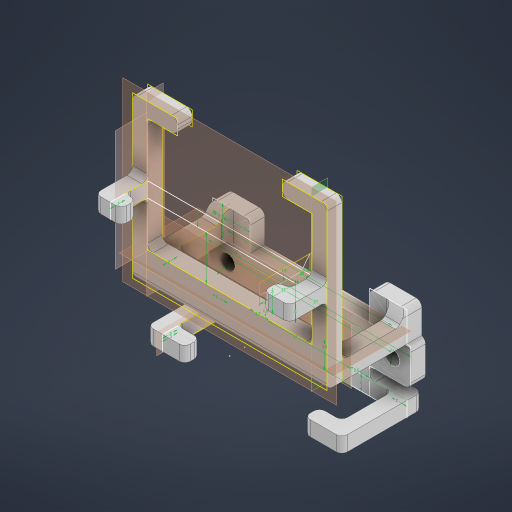
# Autodesk Inventor part: battery-stopper-3
Saved by Autodesk Inventor 2023.5 (Build 275446000, 446)
## iProperties
Created: 2025-02-09
Part Number: battery-stopper-3
Material: 一般
Document SubType Name: Modeling
Designer: IshiiLabHonda
Density: 1 g/cm^3
Appearance: 既定
Author: IshiiLabHonda
Autodesk Inventor part; units mm, degrees
ref_plane "YZ Plane" through (0, 0, 0) normal (1, 0, 0) x (0, 1, 0)
ref_plane "XZ Plane" through (0, 0, 0) normal (0, 1, 0) x (-1, 0, 0)
ref_plane "XY Plane" through (0, 0, 0) normal (0, 0, 1) x (1, 0, 0)
sketch "スケッチ1" plane through (0, 0, 0) normal (0, 0, 1) x (1, 0, 0)
  line L0 (0, 0) -> (0, 1.8035) construction
  line L1 (1.7104, 0) -> (0, 0) construction
  circle A0 centre (-11, 0) radius 1
  circle A1 centre (11, 0) radius 1
  line L2 (-13.5, 2.5) -> (13.5, 2.5)
  line L3 (13.5, 2.5) -> (13.5, -2.5)
  line L4 (13.5, -2.5) -> (-13.5, -2.5)
  line L5 (-13.5, -2.5) -> (-13.5, 2.5)
  line L6 (-13.5, 2.5) -> (13.5, -2.5) construction
  line L7 (13.5, 2.5) -> (-13.5, -2.5) construction
  circle A2 centre (-11, 0) radius 2.5 construction
  line L8 (-13, 6.5) -> (-8, 6.5)
  line L9 (-8, 6.5) -> (-8, 2.5)
  line L10 (-8, 2.5) -> (-13, 2.5)
  line L11 (-13, 2.5) -> (-13, 6.5)
  line L12 (-13, 6.5) -> (-8, 2.5) construction
  line L13 (-8, 6.5) -> (-13, 2.5) construction
  line L14 (-11, 6.5) -> (-11, 2.5)
  line L15 (13, 6.5) -> (8, 6.5)
  line L16 (8, 6.5) -> (8, 2.5)
  line L17 (13, 2.5) -> (13, 6.5)
  line L18 (13, 6.5) -> (8, 2.5) construction
  line L19 (8, 6.5) -> (13, 2.5) construction
  line L20 (11, 6.5) -> (11, 2.5)
  line L21 (-5.5, -2.5) -> (-5.5, -6)
  line L22 (-8, -2.5) -> (-8, -6)
  line L23 (8, -2.5) -> (8, -6)
  line L24 (5.5, -2.5) -> (5.5, -6)
  line L25 (8, -6) -> (5.5, -6)
  line L26 (-5.5, -6) -> (-8, -6)
  line L27 (13, -4) -> (-13, -4)
  line L28 (13, -6) -> (-13, -6)
  line L29 (13, -4) -> (13, -6)
  line L30 (-13, -4) -> (-13, -6)
  line L31 (-11, -4) -> (-11, -6)
  line L32 (11, -4) -> (11, -6)
  point P0 (-10.5, 4.5)
  point P1 (10.5, 4.5)
  point P2 (8, 2.5)
  point P3 (-8, -6)
  point P4 (-5.5, -6)
  point P5 (5.5, -6)
  point P6 (8, -4)
  point P7 (5.5, -4)
  point P8 (-5.5, -4)
  point P9 (-8, -4)
  dimension "d0" = 2
  dimension "d1" = 2
  dimension "d2" = 22
  dimension "d3" = 5
  dimension "d4" = 27
  dimension "d12" = 5
  dimension "d42" = 2
  dimension "d43" = 4
  dimension "d45" = 5
  dimension "d46" = 22
  dimension "d104" = 2.5
  dimension "d105" = 2.5
  dimension "d106" = 11
  dimension "d109" = 3.5
  dimension "d114" = 2
  dimension "d165" = 2
  dimension "d166" = 2
  constraints: 66 end point, 17 point on line, 15 parallel, 8 symmetric about line, 4 midpoint, 3 centre point, 3 coincident, 3 perpendicular, 3 vertical, 1 collinear, 1 other
  measures "d0" diameter of A0
  measures "d1" diameter of A1
  measures "d2" distance of A1.centre A0.centre
  measures "d3" distance between parallel lines of L4 L2
  measures "d4" distance between parallel lines of L3 L5
  measures "d12" diameter of A2
  measures "d42" distance between parallel lines of L11 L14
  measures "d43" distance between parallel lines of L10 L8
  measures "d45" distance between parallel lines of L11 L9
  measures "d46" distance between parallel lines of L20 L14
  measures "d104" distance between parallel lines of L24 L23
  measures "d105" distance between parallel lines of L22 L21
  measures "d106" distance between parallel lines of L21 L24
  measures "d109" distance between parallel lines of L4 L25
  measures "d114" distance between parallel lines of L25 L27
  measures "d165" distance between parallel lines of L30 L31
  measures "d166" distance between parallel lines of L29 L32
extrude "押し出し3" add sketch "スケッチ1" against normal blind 2 contours L2 L3 L4 L5
extrude "押し出し4" add sketch "スケッチ1" against normal blind 2 contours A0 | A1 | L2 L3 L4 L5
extrude "押し出し9" cut sketch "スケッチ1" against normal up to surface (2 mm away) contours A0 | A1
extrude "押し出し11" add sketch "スケッチ1" along normal blind 6.7 contours L11 L8 L14 L2 | L20 L15 L17 L2
extrude "押し出し12" add sketch "スケッチ1" against normal up to surface (2 mm away) contours L11 L8 L14 L2 | L14 L8 L9 L2 | L16 L15 L20 L2 | L20 L15 L17 L2
sketch "スケッチ5" plane through (0, 0, 0) normal (1, 0, 0) x (0, 1, 0)
  line L0 (2.5, 0) -> (-2.5, 0) projected
  line L1 (2.5, 0) -> (2.5, -2) projected
  line L2 (-2.5, -2) -> (2.5, -2) projected
  line L3 (-2.5, 0) -> (-2.5, -2) projected
  line L4 (2.5, 0) -> (2.5, 6.7) projected
  line L5 (6.5, 6.7) -> (2.5, 6.7) projected
  line L6 (6.5, -2) -> (6.5, 6.7) projected
  line L7 (2.5, -2) -> (6.5, -2) projected
  line L8 (2.5, 0) -> (2.5, -2) projected
  line L9 (2.5, 0) -> (6.5, 0) projected
  line L10 (6.5, 0) -> (5, 1.1719)
  line L11 (2.5, 0) -> (2, 0.3906)
  line L12 (5, 1.1719) -> (5, 6.7)
  line L13 (5, 6.7) -> (2, 6.7)
  line L14 (2, 6.7) -> (2, 0.3906)
  point P0 (0, 0)
  dimension "d52" = 3
  dimension "d53" = 1.5
  dimension "d54" = 38
  dimension "d55" = 6.7
  constraints: 10 end point, 2 parallel, 1 collinear, 1 perpendicular
  measures "d52" distance between parallel lines of L12 L14
  measures "d53" distance between parallel lines of L6 L12
  measures "d54" angle of L9 L10
  measures "d55" distance between parallel lines of L9 L13
extrude "押し出し13" cut sketch "スケッチ5" against normal up to surface (13 mm away) contours L10 L12 L5 L6
extrude "押し出し14" cut sketch "スケッチ5" along normal up to surface (13 mm away) contours L10 L12 L5 L6
ref_plane "作業平面2" through (-11, 2.5, 6.7) normal (1, 0, 0) x (0, 0, -1)
sketch "スケッチ6" plane through (-11, 2.5, 6.7) normal (1, 0, 0) x (0, 0, -1)
  line L0 (6.7, 4) -> (5.5281, 2.5) projected
  line L1 (5.5281, 2.5) -> (0, 2.5) projected
  line L2 (0, 0) -> (0, 2.5) projected
  line L3 (6.7, 0) -> (0, 0) projected
  line L4 (6.7, 0) -> (6.7, 4) projected
  line L5 (0, 0) -> (0, 2.5) projected
  line L6 (0, 0) -> (-2, 0)
  line L7 (0, 2.5) -> (-2, 2.5)
  line L8 (-2, 0) -> (-2, 2.5)
  point P0 (6.7, -2.5)
  dimension "d61" = 2
  constraints: 6 end point, 1 collinear, 1 parallel, 1 perpendicular
  measures "d61" distance between parallel lines of L2 L8
extrude "押し出し15" add sketch "スケッチ6" along normal up to surface (24 mm away) contours L2 L6 L8 L7
extrude "押し出し16" add sketch "スケッチ6" against normal up to surface (2 mm away) contours L2 L6 L8 L7
ref_plane "作業平面4" through (-13, 5, 8.7) normal (0, 0, 1) x (1, 0, 0)
extrude "押し出し29" add sketch "スケッチ1" along normal blind 6.7 contours L31 L28 L30 L27 | L27 L29 L28 L32
extrude "押し出し30" add sketch "スケッチ1" against normal blind 2 contours L4 L21 L27 L22 | L27 L21 L26 L22 | L22 L28 L31 L27 | L4 L23 L27 L24 | L27 L24 L28 L21 | L31 L28 L30 L27 | L27 L23 L25 L24 | L27 L32 L28 L23 | L27 L29 L28 L32
ref_plane "作業平面8" through (-11, -6, 0) normal (1, 0, 0) x (0, 0, -1)
sketch "スケッチ13" plane through (-13, 5, 8.7) normal (0, 0, 1) x (1, 0, 0)
  line L0 (26, -2.5) -> (26, 0) projected
  line L1 (26, 0) -> (0, 0) projected
  line L2 (0, 0) -> (0, -2.5) projected
  line L3 (0, -2.5) -> (26, -2.5) projected
  line L4 (24, 1.5) -> (24, -2.5) projected
  line L5 (2, -2.5) -> (2, 0) projected
  point P0 (13, -5)
  point P1 (24, 0)
extrude "押し出し32" add sketch "スケッチ13" along normal blind 2 contours L3 L4 L1 L0 | L3 L2 L1 L5
ref_plane "作業平面9" through (-13, 5, 1.1719) normal (0, 1, 0) x (1, 0, 0)
sketch "スケッチ14" plane through (-13, 5, 1.1719) normal (0, 1, 0) x (1, 0, 0)
  line L0 (2, 0) -> (2, -5.5281) projected
  line L1 (2, 0) -> (0, 0) projected
  line L2 (0, -9.5281) -> (0, 0) projected
  line L3 (2, -9.5281) -> (0, -9.5281) projected
  line L4 (2, -7.5281) -> (2, -9.5281) projected
  line L5 (24, -7.5281) -> (2, -7.5281) projected
  line L6 (24, -7.5281) -> (24, -9.5281) projected
  line L7 (26, -9.5281) -> (24, -9.5281) projected
  line L8 (26, 0) -> (26, -9.5281) projected
  line L9 (24, 0) -> (26, 0) projected
  line L10 (24, -5.5281) -> (24, 0) projected
  line L11 (2, -5.5281) -> (24, -5.5281) projected
  line L12 (24, -7.5281) -> (2, -7.5281) projected
  line L13 (2, -7.5281) -> (0, -7.5281)
  line L14 (0, -9.5281) -> (0, 0) projected
  line L15 (24, -7.5281) -> (26, -7.5281)
  line L16 (26, 0) -> (26, -9.5281) projected
  point P0 (13, 1.1719)
  constraints: 4 end point, 3 point on line, 1 perpendicular
extrude "押し出し33" add sketch "スケッチ14" along normal blind 19 contours L13 L4 L3 L2 | L15 L8 L7 L6
ref_plane "作業平面10" through (11, 2.5, 8.7) normal (-1, 0, 0) x (0, 0, 1)
sketch "スケッチ15" plane through (11, 2.5, 8.7) normal (-1, 0, 0) x (0, 0, 1)
  line L0 (0, 0) -> (0, 2.5) projected
  line L1 (0, 0) -> (2, 0) projected
  line L2 (2, 0) -> (2, 21.5) projected
  line L3 (0, 21.5) -> (2, 21.5) projected
  line L4 (0, 2.5) -> (0, 21.5) projected
  line L5 (2, 19.5) -> (0, 19.5)
  point P0 (-8.7, -2.5)
  dimension "d130" = 2
  constraints: 2 end point, 2 point on line, 1 parallel
  measures "d130" distance between parallel lines of L3 L5
ref_plane "作業平面11" through (-11, 2.5, 10.7) normal (1, 0, 0) x (0, 0, -1)
sketch "スケッチ16" plane through (-11, 2.5, 10.7) normal (1, 0, 0) x (0, 0, -1)
  line L0 (2, 2.5) -> (2, 0) projected
  line L1 (2, 2.5) -> (2, 21.5) projected
  line L2 (0, 21.5) -> (2, 21.5) projected
  line L3 (0, 0) -> (0, 21.5) projected
  line L4 (2, 0) -> (0, 0) projected
  line L5 (0, 19.5) -> (2, 19.5)
  line L6 (0, 21.5) -> (2, 21.5) projected
  point P0 (10.7, -2.5)
  dimension "d132" = 2
  constraints: 2 end point, 2 point on line, 1 parallel
  measures "d132" distance between parallel lines of L2 L5
extrude "押し出し34" add sketch "スケッチ15" along normal blind 4 contours L4 L3 L2 L5
extrude "押し出し35" add sketch "スケッチ16" along normal blind 4 contours L5 L3 L2 L1
sketch "スケッチ19" plane through (-13, 5, 8.7) normal (0, 0, 1) x (1, 0, 0)
  line L0 (2, 0) -> (2, -2.5) projected
  line L1 (2, -2.5) -> (24, -2.5) projected
  line L2 (24, -2.5) -> (24, 0) projected
  line L3 (24, 0) -> (2, 0) projected
  line L4 (0, -2.5) -> (2, -2.5) projected
  line L5 (2, -2.5) -> (2, 17) projected
  line L6 (2, 17) -> (6, 17) projected
  line L7 (6, 19) -> (6, 17) projected
  line L8 (0, 19) -> (6, 19) projected
  line L9 (0, -2.5) -> (0, 19) projected
  line L10 (24, -2.5) -> (24, 17) projected
  line L11 (24, -2.5) -> (26, -2.5) projected
  line L12 (26, -2.5) -> (26, 19) projected
  line L13 (26, 19) -> (20, 19) projected
  line L14 (20, 17) -> (20, 19) projected
  line L15 (24, 17) -> (20, 17) projected
  line L16 (24, 1.8) -> (2, 1.8)
  line L17 (24, 0) -> (2, 0) projected
  point P0 (13, -5)
  dimension "d144" = 1.8
  constraints: 2 end point, 2 point on line, 1 parallel, 1 perpendicular
  measures "d144" distance between parallel lines of L3 L16
extrude "押し出し38" add sketch "スケッチ19" along normal up to surface (2 mm away) contours L3 L2 L1 L0 | L5 L16 L10 L3
ref_plane "作業平面12" through (-13, 5, 10.7) normal (0, 0, 1) x (1, 0, 0)
sketch "スケッチ20" plane through (-13, 5, 10.7) normal (0, 0, 1) x (1, 0, 0)
  line L0 (0, -2.5) -> (26, -2.5) projected
  line L1 (26, -2.5) -> (26, 19) projected
  line L2 (26, 19) -> (20, 19) projected
  line L3 (20, 17) -> (20, 19) projected
  line L4 (24, 17) -> (20, 17) projected
  line L5 (24, 1.8) -> (24, 17) projected
  line L6 (2, 1.8) -> (24, 1.8) projected
  line L7 (2, 1.8) -> (2, 17) projected
  line L8 (2, 17) -> (6, 17) projected
  line L9 (6, 19) -> (6, 17) projected
  line L10 (0, 19) -> (6, 19) projected
  line L11 (0, -2.5) -> (0, 19) projected
  line L12 (0, 9.8) -> (26, 9.8)
  line L13 (0, 7.8) -> (26, 7.8)
  line L14 (2, 1.8) -> (2, 17) projected
  point P0 (13, -5)
  point P1 (24, 7.8)
  point P2 (24, 9.8)
  point P3 (2, 7.8)
  point P4 (2, 9.8)
  dimension "d148" = 2
  dimension "d163" = 6
  constraints: 4 end point, 4 point on line, 2 perpendicular
  measures "d148" distance between parallel lines of L13 L12
  measures "d163" distance between parallel lines of L6 L13
extrude "押し出し39" add sketch "スケッチ20" along normal blind 3 contours L11 L12 L7 L13 | L13 L5 L12 L1
ref_plane "作業平面13" through (-11, 22, 10.7) normal (1, 0, 0) x (0, 0, -1)
sketch "スケッチ21" plane through (-11, 22, 10.7) normal (1, 0, 0) x (0, 0, -1)
  line L0 (0, -15.2) -> (2, -15.2) projected
  line L1 (2, -15.2) -> (2, 0) projected
  line L2 (2, 0) -> (0, 0) projected
  line L3 (0, -7.2) -> (0, 0) projected
  line L4 (0, -7.2) -> (-3, -7.2) projected
  line L5 (-3, -9.2) -> (-3, -7.2) projected
  line L6 (0, -9.2) -> (-3, -9.2) projected
  line L7 (0, -15.2) -> (0, -9.2) projected
  line L8 (0, -9.2) -> (-3, -9.2) projected
  line L9 (-3, -9.2) -> (-5, -9.2)
  line L10 (-5, -9.2) -> (-5, -7.2)
  line L11 (-5, -7.2) -> (-3, -7.2)
  point P0 (10.7, -22)
  dimension "d152" = 2
  constraints: 6 end point, 2 perpendicular, 1 horizontal
  measures "d152" distance between parallel lines of L5 L10
extrude "押し出し40" add sketch "スケッチ21" along normal blind 1.5 contours L9 L10 L11 L5
extrude "押し出し41" add sketch "スケッチ21" against normal up to surface (2 mm away) contours L9 L10 L11 L5
mirror "ミラー1" about plane through (0, 0, 0) normal (1, 0, 0) of "押し出し41", "押し出し40"
sketch "スケッチ22" plane through (-11, -6, 0) normal (1, 0, 0) x (0, 0, -1)
  line L0 (2, 2) -> (-6.7, 2) projected
  line L1 (0, 0) -> (0, 2) projected
  line L2 (0, 2) -> (-6.7, 2) projected
  line L3 (-6.7, 0) -> (-6.7, 2) projected
  line L4 (0, 0) -> (-6.7, 0) projected
  line L5 (-6.7, 0) -> (-6.7, 2) projected
  line L6 (-6.7, 0) -> (-8.7, 0)
  line L7 (-8.7, 0) -> (-8.7, 2)
  line L8 (-8.7, 2) -> (-6.7, 2)
  line L9 (-6.7, 0) -> (-6.7, 2)
  point P0 (0, 6)
  point P1 (-6.7, 2)
  dimension "d157" = 2
  dimension "d158" = 2
  constraints: 8 end point, 2 parallel, 2 perpendicular, 2 point on line
  measures "d157" distance between parallel lines of L3 L7
  measures "d158" distance between parallel lines of L9 L7
extrude "押し出し42" add sketch "スケッチ22" along normal blind 3 contours L3 L6 L7 L8
extrude "押し出し43" add sketch "スケッチ22" against normal up to surface (2 mm away) contours L3 L6 L7 L8
mirror "ミラー2" about plane through (0, 0, 0) normal (1, 0, 0) of "押し出し43", "押し出し42"
fillet "フィレット1" radius 0.75 10 edges at (11, 4.5, 0) (-11, 4.5, 0) (-11, -5, 0) (11, -5, 0) (11, -5, 6.7) (-11, -5, 6.7) (11, 3.75, 6.7) (-11, 3.75, 6.7) (-11, 13.8, 13.7) (11, 13.8, 13.7)
fillet "フィレット2" radius 0.75 12 edges at (9.5, 13.8, 13.7) (9.5, 13.8, 15.7) (13, 13.8, 15.7) (-9.5, 13.8, 13.7) (-9.5, 13.8, 15.7) (-13, 13.8, 15.7) (-8, -5, 8.7) (-8, -5, 6.7) (-13, -5, 8.7) (8, -5, 8.7) (8, -5, 6.7) (13, -5, 8.7)
fillet "フィレット3" radius 0.75 17 edges at (-7, 22, 9.7) (-7, 24, 9.7) (7, 22, 9.7) (7, 24, 9.7) (-11, 22, 9.7) (-11, 6.8, 9.7) (11, 6.8, 9.7) (-13, 24, 9.7) (13, 24, 9.7) (-5.5, -2.5, -1) (-5.5, -4, -1) (5.5, -2.5, -1) (5.5, -4, -1) (8, -4, -1) (8, -2.5, -1) (-8, -2.5, -1) (-8, -4, -1)
fillet "フィレット4" radius 0.75 8 edges at (-13.5, 2.5, -1) (-13.5, -2.5, -1) (13.5, 2.5, -1) (13.5, -2.5, -1) (-13, 6.5, -1) (-8, 6.5, -1) (8, 6.5, -1) (13, 6.5, -1)
fillet "フィレット5" radius 0.75 4 edges at (-12, 12.8, 10.7) (-12, 14.8, 10.7) (12, 14.8, 10.7) (12, 12.8, 10.7)
fillet "フィレット6" radius 0.75 1 edges at (0, 5, 8.7)
fillet "フィレット7" radius 0.75 1 edges at (0, 2.5, 10.7)
fillet "フィレット8" radius 0.4 2 edges at (-11.625, 2.5, 0) (11.625, 2.5, 0)
fillet "フィレット9" radius 0.75 2 edges at (12, 5, 1.1719) (-12, 5, 1.1719)
fillet "フィレット10" radius 0.75 2 edges at (-13, -5, -2) (13, -5, -2)
